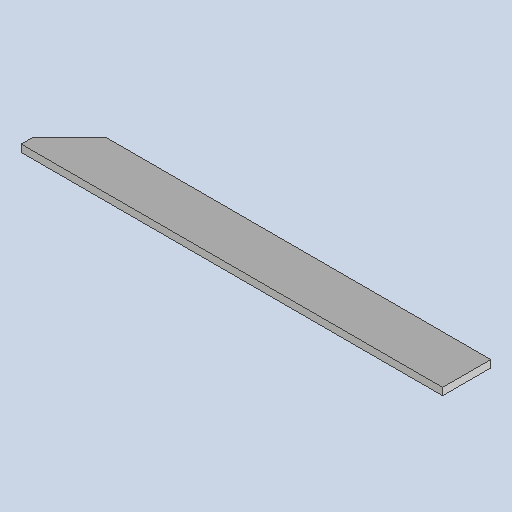
# Autodesk Inventor part: MSC 406 FLANGE COVER PLATE 500
Saved by Autodesk Inventor 2025 (Build 290162010, 162A)
## iProperties
Created: 2024-06-25
Part Number: MSC 406 FLANGE COVER PLATE 500
Material: Stainless Steel
Document SubType Name: Sheet Metal
Designer: pokla
Density: 8 g/cm^3
Sheet Metal Rule: AISI304 3mm Die 32
Appearance: Default
Flat Pattern Width: 2 cm
Flat Pattern Length: 17.5 cm
Flat Pattern Area: 35 cm^2
Sheet Metal Width: 20,000 mm
Sheet Metal Length: 175,000 mm
Sheet Metal Area: 3500,000 mm^2
Stock Number: МОО 406 усилитель крышки фланца 500 пластина
Mass: 81.3 g
Surface Area: 79.1864 cm^2
Volume: 10.1625 cm^3
Author: pokla
Autodesk Inventor part; units mm, degrees
ref_plane "YZ Plane" through (0, 0, 0) normal (1, 0, 0) x (0, 1, 0)
ref_plane "XZ Plane" through (0, 0, 0) normal (0, 1, 0) x (-1, 0, 0)
ref_plane "XY Plane" through (0, 0, 0) normal (0, 0, 1) x (1, 0, 0)
sketch "Sketch1" plane through (0, 0, 0) normal (0, 0, 1) x (1, 0, 0)
  line L0 (-175, 20) -> (0, 20)
  line L1 (0, 20) -> (0, 0)
  line L2 (0, 0) -> (-175, 0)
  line L3 (-175, 0) -> (-175, 20)
  dimension "d2" = 20
  dimension "d3" = 175
  measures "d2" distance of L0.end L1.end
  measures "d3" distance of L1.end L2.end
extrude "Plate1" add sketch "Sketch1" along normal mid plane 3
chamfer "Chamfer1" distance 15 angle 45 1 edges at (-175, 20, 0)
equation "\"d4\" = Thickness"
equation "\"BendReliefWidth\" = Thickness"
equation "\"BendReliefDepth\" = 0.5 * Thickness"
equation "\"CornerReliefSize\" = 4 * Thickness"
equation "\"MinimumRemnant\" = 2 * Thickness"
equation "\"TransitionRadius\" = BendRadius"
equation "\"JacobiRadiusSize\" = BendRadius"
equation "\"GapSize\" = Thickness"
equation "\"Thickness\" = 3"
equation "\"BendRadius\" = 5"
body "Solid1"
